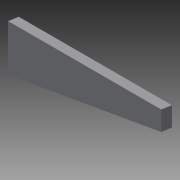
# Autodesk Inventor part: Panel_side
Saved by Autodesk Inventor 2013 (Build 170138000, 138)
## iProperties
Created: 2012-08-20
Part Number: Panel_side
Material: Generic
Document SubType Name: Modeling
Designer: Brandon
Density: 1 g/cm^3
d0: 100.00 deg
d1: 25.500 mm
d5: 203.085 mm
d7: 12.000 mm
d8: 0.00 deg
d12: 10.00 deg
d13: -10.00 deg
Author: Brandon
Autodesk Inventor part; units mm, degrees
ref_plane "Work Plane1" through (99.4266, 0, -12.9365) normal (0.9848078, -0.1736482, 0) x (0, 0, -1)
ref_plane "Work Plane2" through (-102.6005, 6, 0) normal (0, 0, 1) x (1, 0, 0)
ref_plane "Work Plane3" through (-101.5425, 12, -61.3094) normal (0.1735668, -0.0306045, -0.9843464) x (0.9848078, 0, 0.1736482)
sketch "Sketch1" plane through (0, 0, 0) normal (0, 1, 0) x (-1, 0, 0)
  line L0 (101.5425, -61.3094) -> (101.5425, 0)
  line L1 (101.5425, 0) -> (-101.5425, 0)
  line L2 (-101.5425, 0) -> (-101.5425, -25.5)
  line L3 (-101.5425, -25.5) -> (101.5425, -61.3094)
  point P0 (0, 0)
  point P1 (0, 0)
  dimension "d0" = 100
  dimension "d1" = 25.5
  dimension "d5" = 203.085
  dimension "d15" = 25.5
  dimension "d16" = 156.1695
  constraints: 8 end point, 2 coincident, 1 midpoint, 1 parallel, 1 perpendicular, 1 vertical
  measures "d0" angle of L2 L3
  measures "d1" distance of L1.end L2.end
  measures "d5" distance of L0.end L1.end
extrude "Extrusion1" add sketch "Sketch1" along normal blind 12
draft "FaceDraft2" angle 10 pull direction (0, -1, 0) faces at (101.5425, 4, -8.5) fixed edges at (101.5425, 12, -12.75)
draft "FaceDraft3" angle -10 pull direction (0, -1, 0) faces at (-101.5425, 4, -40.8729) fixed edges at (-101.5425, 12, -30.6547)
equation "\"d15\" = d1"
body "Solid1"
